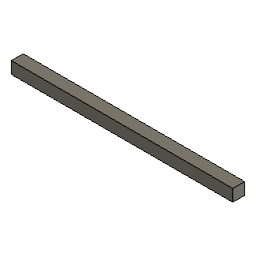
平行于丝杆的定位小杆 (Autodesk Fusion 360 design; units mm, degrees)
part number: 2026-08-06-20-04-20-174
Autodesk Fusion 360 part; units mm, degrees
sketch "草图1" plane through (0, 0, 0) normal (0, 1, 0) x (1, 0, 0)
  line L0 (-100, 50) -> (-7.8, 50)
  line L1 (-7.8, 50) -> (-7.8, 45)
  line L2 (-7.8, 45) -> (-100, 45)
  line L3 (-100, 45) -> (-100, 50)
  dimension "d1" = 92.2
  dimension "d2" = 5
  constraint horizontal L0
  constraint vertical L1
  constraint horizontal L2
  constraint vertical L3
  measures "d1" distance of L0.start L0.end
  measures "d2" distance of L0.start L2.end
extrude "拉伸1" add sketch "草图1" along normal blind 5
